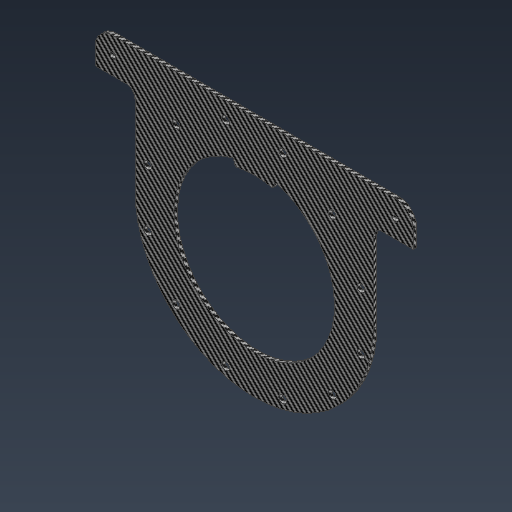
# Autodesk Inventor part: base4
Saved by Autodesk Inventor 2021 (Build 250183000, 183)
## iProperties
Created: 2021-07-20
Part Number: base4
Material: CFRP
Document SubType Name: Sheet Metal
Designer: yuta0
Density: 1.43 g/cm^3
Sheet Metal Rule: Default_mm
Appearance: カーボンファイバー
購入先: カーボン
在庫数: 0.0
Author: yuta0
Autodesk Inventor part; units mm, degrees
ref_plane "YZ Plane" through (0, 0, 0) normal (1, 0, 0) x (0, 1, 0)
ref_plane "XZ Plane" through (0, 0, 0) normal (0, 1, 0) x (-1, 0, 0)
ref_plane "XY Plane" through (0, 0, 0) normal (0, 0, 1) x (1, 0, 0)
sketch "スケッチ1" plane through (0, 0, 0) normal (0, 0, 1) x (1, 0, 0)
  line L0 (-90, -67.5) -> (90, -67.5)
  line L1 (90, -67.5) -> (90, 70)
  line L2 (90, 70) -> (-90, 70)
  line L3 (-90, 70) -> (-90, -67.5)
  point P0 (0, 0)
  point P1 (-29.0861, -67.5)
  dimension "d37" = 90
  dimension "d38" = 70
  dimension "d40" = 90
  dimension "d41" = 67.5
  constraints: 8 end point, 2 parallel, 1 horizontal, 1 perpendicular, 1 point on line
  measures "d37" distance from line of L1 point (0, 0)
  measures "d38" distance from line of point (0, 0) L2
  measures "d40" distance from line of point (0, 0) L3
  measures "d41" distance from line of point (0, 0) L0
extrude "プレート1" add sketch "スケッチ1" along normal blind 2
sketch "スケッチ2" plane through (0, 0, 2) normal (0, 0, 1) x (1, 0, 0)
  circle A0 centre (0, 0) radius 45.5
  dimension "d5" = 91
  constraints: 1 centre point, 1 coincident
  measures "d5" diameter of A0
extrude "押し出し1" cut sketch "スケッチ2" against normal blind 10
sketch "スケッチ3" plane through (0, 0, 2) normal (0, 0, 1) x (1, 0, 0)
  circle A0 centre (0, 0) radius 62.5
  point P0 (-16.1762, 60.3704)
  point P1 (-44.1942, 44.1942)
  point P2 (-60.3704, 16.1762)
  point P3 (-60.3704, -16.1762)
  point P4 (-44.1942, -44.1942)
  point P5 (-16.1762, -60.3704)
  point P6 (16.1762, -60.3704)
  point P7 (44.1942, -44.1942)
  point P8 (60.3704, -16.1762)
  point P9 (60.3704, 16.1762)
  point P10 (44.1942, 44.1942)
  point P11 (16.1762, 60.3704)
  dimension "d8" = 125
  dimension "d11" = 360
  dimension "d20" = 0
  constraints: 1 coincident, 16 other
  measures "d20" vertical distance of point (16.176, 60.37) point (-16.176, 60.37)
hole "穴1" at (-16.1762, 60.3704, 2) at (-44.1942, 44.1942, 2) at (-60.3704, 16.1762, 2) at (-60.3704, -16.1762, 2) at (-44.1942, -44.1942, 2) at (-16.1762, -60.3704, 2) at (16.1762, -60.3704, 2) at (44.1942, -44.1942, 2) at (60.3704, -16.1762, 2) at (60.3704, 16.1762, 2) at (44.1942, 44.1942, 2) at (16.1762, 60.3704, 2) direction (0, 0, -1) diameter 4.5 end through all clearance for "Flat Head Machine Screw" size "M4" standard "Ansi Metric M Profile"
fillet "コーナーR2" radius 10 2 edges at (-90, 70, 1) (90, 70, 1)
sketch "スケッチ5" plane through (0, 0, 2) normal (0, 0, 1) x (1, 0, 0)
  arc A0 (-80, 70) -> (-90, 60) centre (-80, 60) ccw projected
  arc A1 (90, 60) -> (80, 70) centre (80, 60) ccw projected
  point P0 (0, 0)
hole "穴2" at (-80, 60, 2) at (80, 60, 2) direction (0, 0, -1) diameter 3.4 end through all clearance for "Socket Head Cap Screw" size "M3" standard "Ansi Metric M Profile"
sketch "スケッチ7" plane through (0, 0, 2) normal (0, 0, 1) x (1, 0, 0)
  circle A0 centre (0, 0) radius 45.5 projected
  circle A1 centre (0, 0) radius 67.5
  line L0 (90, -67.5) -> (-90, -67.5) projected
  line L1 (-90, -67.5) -> (-90, 60) projected
  line L2 (-90, -67.5) -> (-67.5, -67.5)
  line L3 (-67.5, -67.5) -> (-67.5, 50)
  line L4 (-67.5, 50) -> (-90, 50)
  line L5 (-90, 50) -> (-90, -67.5)
  line L6 (90, -67.5) -> (67.5, -67.5)
  line L7 (67.5, -67.5) -> (67.5, 50)
  line L8 (67.5, 50) -> (90, 50)
  line L9 (90, 50) -> (90, -67.5)
  line L10 (-80, 70) -> (80, 70) projected
  point P0 (67.5, 0)
  point P1 (0, -67.5)
  point P2 (-67.5, 0)
  dimension "d56" = 20
  dimension "d57" = 20
  constraints: 16 end point, 4 parallel, 3 tangent, 2 horizontal, 2 perpendicular, 1 centre point, 1 coincident
  measures "d56" distance between parallel lines of L10 L4
  measures "d57" distance between parallel lines of L10 L8
extrude "押し出し4" cut sketch "スケッチ7" against normal blind 10 contours L7 L0 A1 | L7 L8 L9 L0 | A1 L0 L3 | L3 L0 L1 L4
fillet "コーナーR4" radius 5 2 edges at (-67.5, 50, 1) (67.5, 50, 1)
sketch "スケッチ9" plane through (0, 0, 2) normal (0, 0, 1) x (1, 0, 0)
  circle A0 centre (0, 0) radius 45.5 projected
  circle A1 centre (0, 0) radius 41.5
  line L0 (0, 0) -> (-11.7763, 43.9496)
  line L1 (11.7763, 43.9496) -> (0, 0)
  line L2 (0, 97.5) -> (0, -95) projected
  point P0 (-10.741, 40.0859)
  point P1 (10.741, 40.0859)
  dimension "d76" = 4
  dimension "d77" = 15
  dimension "d78" = 15
  constraints: 4 end point, 2 point on circle, 1 centre point
  measures "d76" radial gap between concentric circles of A0 A1
  measures "d77" angle of L2 L0
  measures "d78" angle of L2 L1
extrude "押し出し5" add sketch "スケッチ9" against normal up to surface (2 mm away) contours L1 A1 L2 A0 | L2 A1 L0 A0 picked at (5.1612, 43.8259) picked at (-6.3577, 43.6684)
fillet "コーナーR5" radius 1 4 edges at (10.741, 40.0859, 1) (-10.741, 40.0859, 1) (-11.7763, 43.9496, 1) (11.7763, 43.9496, 1)
equation "\"d40\" = d37"
equation "\"d18\" = Thickness"
equation "\"d47\" = Thickness"
equation "\"d2\" = Thickness"
equation "\"BendRadius\" = Thickness"
equation "\"BendReliefWidth\" = Thickness"
equation "\"BendReliefDepth\" = 0.5 * Thickness"
equation "\"CornerReliefSize\" = 4 * Thickness"
equation "\"MinimumRemnant\" = 2 * Thickness"
equation "\"TransitionRadius\" = BendRadius"
equation "\"JacobiRadiusSize\" = BendRadius"
equation "\"GapSize\" = Thickness"
equation "\"Thickness\" = 2"
